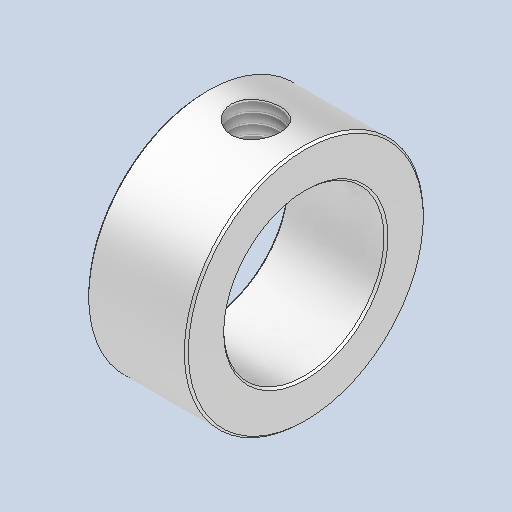
# Autodesk Inventor part: pos-ring_d8_D12_t5_M3_V1
Saved by Autodesk Inventor 2023 (Build 270158000, 158)
## iProperties
Created: 2023-02-13
Part Number: pos-ring_d8_D12_t5_M3_V1
Material: Messing, weicher Gelbton
Document SubType Name: Modeling
Designer: Mathi
Density: 8.47 g/cm^3
Appearance: Messing - satiniert
Author: Mathi
Autodesk Inventor part; units mm, degrees
note: some values were not read from the file. Chosen so that the rebuilt part matches the saved one: direction of "Bohrung1".
ref_plane "YZ Plane" through (0, 0, 0) normal (1, 0, 0) x (0, 1, 0)
ref_plane "XY Plane" through (0, 0, 0) normal (0, 0, 1) x (1, 0, 0)
sketch "Skizze1" plane through (0, 0, 0) normal (0, 0, 1) x (1, 0, 0)
  line L0 (-9.8448, 0) -> (9.4061, 0)
  line L1 (-2.4, 4.025) -> (2.4, 4.025)
  line L2 (2.5, 4.125) -> (2.5, 5.9)
  line L3 (2.4, 6) -> (-2.4, 6)
  line L4 (-2.5, 5.9) -> (-2.5, 4.125)
  line L5 (0, 0) -> (0, 4.025) construction
  line L6 (-2.4, 4.025) -> (-2.5, 4.125)
  line L7 (2.4, 4.025) -> (2.5, 4.125)
  line L8 (2.5, 5.9) -> (2.4, 6)
  line L9 (-2.4, 6) -> (-2.5, 5.9)
  point P0 (-2.5, 4.025)
  point P1 (2.5, 6)
  point P2 (2.5, 4.025)
  point P3 (-2.5, 6)
  dimension "d0" = 0.1
  dimension "d1" = 0.1
  dimension "d2" = 0.1
  dimension "d3" = 0.1
  dimension "d4" = 0.1
  dimension "d5" = 0.1
  dimension "d6" = 0.1
  dimension "d7" = 0.1
  dimension "d8" = 8.05
  dimension "d9" = 12
  dimension "d10" = 5
  constraints: 20 end point, 9 point on line, 2 horizontal, 2 parallel, 1 midpoint, 1 perpendicular, 1 vertical
  measures "d0" distance of L1.start point (-2.5, 4.025)
  measures "d1" distance of L4.end point (-2.5, 4.025)
  measures "d2" distance of L1.end point (2.5, 4.025)
  measures "d3" distance of L2.start point (2.5, 4.025)
  measures "d4" distance of L2.end point (2.5, 6)
  measures "d5" distance of L3.start point (2.5, 6)
  measures "d6" distance of L3.end point (-2.5, 6)
  measures "d7" distance of L4.start point (-2.5, 6)
  measures "d8" diameter of L1 L0
  measures "d9" diameter of L3 L0
  measures "d10" distance between parallel lines of L2 L4
revolve "Umdrehung1" add sketch "Skizze1" angle 360 about axis through (-9.8448, 0, 0) along (1, 0, 0)
ref_plane "Arbeitsebene1" through (0, 6, 0) normal (0, 1, 0) x (-1, 0, 0)
sketch "Skizze2" plane through (0, 6, 0) normal (0, 1, 0) x (-1, 0, 0)
  point P0 (0, 0)
  point P1 (0, 0)
  constraints: 1 coincident
hole "Bohrung1" at (0, 6, 0) direction (0, -1, 0) diameter 2.459 end up to surface thread size "M3x0.5" class "6H" standard "ANSI Metric M Profile"
equation "\"d1\" = d0"
equation "\"d2\" = d0"
equation "\"d3\" = d2"
equation "\"d4\" = d0"
equation "\"d5\" = d4"
equation "\"d6\" = d0"
equation "\"d7\" = d6"
